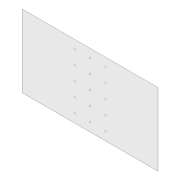
# Autodesk Inventor part: GE-12095
Saved by Autodesk Inventor 2012 (Build 160160000, 160)
## iProperties
Created: 2011-10-27
Part Number: GE-12095
Document SubType Name: Modeling
Designer: dfoster
Density: 1 g/cm^3
Description: Bridge Surface
Mass: 8441.57 g
Surface Area: 53435.7 cm^2
Volume: 8441.57 cm^3
Material: Default
Title: Bridge Surface
Author: dfoster
Autodesk Inventor part; units mm, degrees
ref_plane "YZ Plane" through (0, 0, 0) normal (1, 0, 0) x (0, 1, 0)
ref_plane "XZ Plane" through (0, 0, 0) normal (0, 1, 0) x (-1, 0, 0)
ref_plane "XY Plane" through (0, 0, 0) normal (0, 0, 1) x (1, 0, 0)
sketch "Sketch1" plane through (0, 0, 0) normal (0, 0, 1) x (1, 0, 0)
  line L0 (0, 0) -> (-2235.2, 0)
  line L1 (-2235.2, 0) -> (-2235.2, -1193.8)
  line L2 (-2235.2, -1193.8) -> (0, -1193.8)
  line L3 (0, -1193.8) -> (0, 0)
  dimension "d0" = 2235.2
  dimension "d1" = 1193.8
  constraints: 8 end point, 2 parallel, 1 horizontal, 1 perpendicular
  measures "d0" distance of L1.end L2.end
  measures "d1" distance of L0.end L1.end
extrude "Extrusion1" add sketch "Sketch1" along normal blind 3.175
sketch "Sketch2" plane through (0, 0, 3.175) normal (0, 0, 1) x (1, 0, 0)
  line L0 (-2235.2, 0) -> (0, 0) projected
  line L1 (-2235.2, -1193.8) -> (-2235.2, 0) projected
  circle A0 centre (-1117.6, -139.7) radius 14.2875
  circle A1 centre (-1117.6, -139.7) radius 101.6
  circle A2 centre (-1117.6, -368.3) radius 14.2875
  circle A3 centre (-1117.6, -368.3) radius 101.6
  circle A4 centre (-1117.6, -596.9) radius 14.2875
  circle A5 centre (-1117.6, -596.9) radius 101.6
  circle A6 centre (-1117.6, -825.5) radius 14.2875
  circle A7 centre (-1117.6, -825.5) radius 101.6
  circle A8 centre (-1117.6, -1054.1) radius 14.2875
  circle A9 centre (-1117.6, -1054.1) radius 101.6
  dimension "d4" = 28.575
  dimension "d5" = 203.2
  dimension "d6" = 1117.6
  dimension "d11" = 139.7
  dimension "d14" = 228.6
  constraints: 10 centre point, 5 coincident, 1 vertical, 16 other
  measures "d4" diameter of A0
  measures "d5" diameter of A1
  measures "d6" distance from line of A0.centre L1
  measures "d11" distance from line of A0.centre L0
  measures "d14" distance of A0.centre A2.centre
extrude "Extrusion2" cut sketch "Sketch2" against normal blind 3.175 contours A0 | A2 | A4 | A6 | A8
pattern_linear "Rectangular Pattern1" count 2 spacing 254 along (1, 0, 0) of "Extrusion2"
pattern_linear "Rectangular Pattern2" count 2 spacing 254 along (-1, 0, 0) of "Extrusion2"
body "Solid1"
